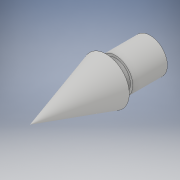
# Autodesk Inventor part: Pencil Tip
Saved by Autodesk Inventor 2018 (Build 220112000, 112)
## iProperties
Created: 2020-01-09
Part Number: Pencil Tip
Material: Generic
Document SubType Name: Modeling
Designer: AOFUser
Density: 1 g/cm^3
Appearance: Default
Author: AOFUser
Autodesk Inventor part; units mm, degrees
ref_plane "YZ Plane" through (0, 0, 0) normal (1, 0, 0) x (0, 1, 0)
ref_plane "XZ Plane" through (0, 0, 0) normal (0, 1, 0) x (-1, 0, 0)
ref_plane "XY Plane" through (0, 0, 0) normal (0, 0, 1) x (1, 0, 0)
sketch "Sketch1" plane through (0, 0, 0) normal (0, 1, 0) x (-1, 0, 0)
  line L0 (0, 0) -> (0, -8.382)
  line L1 (0, -8.382) -> (0, -9.398)
  line L2 (0, -9.398) -> (0, -13.208)
  line L3 (0, -8.382) -> (2.54, -8.382)
  line L4 (2.54, -8.382) -> (0, 0)
  line L5 (0, -9.398) -> (1.651, -9.398)
  line L6 (1.651, -9.398) -> (1.651, -8.382)
  line L7 (0, -13.208) -> (1.905, -13.208)
  line L8 (1.905, -13.208) -> (1.905, -9.398)
  line L9 (1.905, -9.398) -> (1.651, -9.398)
  line L10 (0, 0) -> (0, -1.016)
  line L11 (1.651, -8.382) -> (1.397, -8.382)
  line L12 (0, -1.016) -> (1.397, -8.382)
  line L13 (1.397, -8.382) -> (1.397, -13.208)
  dimension "d0" = 8.382
  dimension "d1" = 1.016
  dimension "d2" = 3.81
  dimension "d3" = 2.54
  dimension "d4" = 1.651
  dimension "d5" = 1.905
  dimension "d6" = 1.016
  dimension "d7" = 0.254
  constraints: 28 end point, 5 perpendicular, 5 point on line, 2 horizontal, 2 vertical
  measures "d0" distance of L0.start L0.end
  measures "d1" distance of L0.end L1.end
  measures "d2" distance of L1.end L2.end
  measures "d3" distance of L0.end L3.end
  measures "d4" distance of L1.end L5.end
  measures "d5" distance of L2.end L7.end
  measures "d6" distance of L0.start L10.end
  measures "d7" distance of L6.end L11.end
revolve "Revolution1" add sketch "Sketch1" angle 360 about axis through (0, 0, 0) along (0, 0, -1) contours L4 L3 L12 L0 | L3 L6 L5 L13 | L5 L9 L8 L7 L13
body "Solid1"
